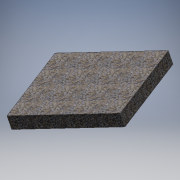
# Autodesk Inventor part: BaseMini
Saved by Autodesk Inventor 2016 (Build 200138000, 138)
## iProperties
Created: 2015-08-01
Part Number: BaseMini
Material: Concrete
Document SubType Name: Modeling
Designer: myhome
Density: 2.40731 g/cm^3
Appearance: Exposed Aggregate - Coarse
Mass: 134809 g
Surface Area: 14200 cm^2
Volume: 56000 cm^3
Author: myhome
Autodesk Inventor part; units mm, degrees
ref_plane "YZ Plane" through (0, 0, 0) normal (1, 0, 0) x (0, 1, 0)
ref_plane "XZ Plane" through (0, 0, 0) normal (0, 1, 0) x (-1, 0, 0)
ref_plane "XY Plane" through (0, 0, 0) normal (0, 0, 1) x (1, 0, 0)
sketch "Sketch5" plane through (0, 0, 0) normal (0, 0, 1) x (1, 0, 0)
  line L0 (0, 0) -> (800, 0)
  line L1 (800, 0) -> (800, 700)
  line L2 (800, 700) -> (0, 700)
  line L3 (0, 700) -> (0, 0)
  line L4 (800, 0) -> (800, 100)
  line L5 (800, 0) -> (800, 20)
  line L6 (800, 20) -> (800, 120)
  line L7 (800, 120) -> (700, 120) construction
  line L8 (700, 120) -> (700, 20) construction
  line L9 (700, 20) -> (800, 20) construction
  line L10 (0, 0) -> (0, 20) construction
  line L11 (0, 20) -> (0, 120) construction
  line L12 (0, 120) -> (100, 120) construction
  line L13 (100, 120) -> (100, 20) construction
  line L14 (100, 20) -> (0, 20) construction
  line L15 (0, 700) -> (0, 680) construction
  line L16 (0, 680) -> (100, 680) construction
  line L17 (100, 680) -> (100, 580) construction
  line L18 (100, 580) -> (0, 580) construction
  line L19 (0, 580) -> (0, 680) construction
  line L20 (800, 700) -> (800, 680) construction
  line L21 (800, 680) -> (700, 680) construction
  line L22 (700, 680) -> (700, 580) construction
  line L23 (700, 580) -> (800, 580) construction
  circle A0 centre (50, 70) radius 50
  circle A1 centre (750, 70) radius 50
  circle A2 centre (50, 630) radius 50
  circle A3 centre (750, 630) radius 50
  dimension "d12" = 800
  dimension "d13" = 700
  dimension "d18" = 20
  dimension "d19" = 100
  dimension "d20" = 100
  dimension "d21" = 100
  dimension "d22" = 100
  dimension "d23" = 20
  dimension "d24" = 100
  dimension "d25" = 100
  dimension "d26" = 100
  dimension "d27" = 100
  dimension "d28" = 20
  dimension "d29" = 100
  dimension "d30" = 100
  dimension "d31" = 100
  dimension "d32" = 100
  dimension "d33" = 20
  dimension "d34" = 100
  dimension "d35" = 100
  dimension "d36" = 100
  constraints: 48 end point, 9 perpendicular, 9 point on line, 4 centre point, 3 parallel, 1 horizontal
  measures "d12" distance of L1.end L2.end
  measures "d13" distance of L0.end L1.end
  measures "d18" distance of L0.end L5.end
  measures "d19" distance of L5.end L6.end
  measures "d20" distance of L6.end L7.end
  measures "d21" distance of L7.end L8.end
  measures "d22" distance of L8.end L5.end
  measures "d23" distance of L0.start L10.end
  measures "d24" distance of L10.end L11.end
  measures "d25" distance of L11.end L12.end
  measures "d26" distance of L12.end L13.end
  measures "d27" distance of L13.end L10.end
  measures "d28" distance of L2.end L15.end
  measures "d29" distance of L15.end L16.end
  measures "d30" distance of L16.end L17.end
  measures "d31" distance of L17.end L18.end
  measures "d32" distance of L18.end L15.end
  measures "d33" distance of L1.end L20.end
  measures "d34" distance of L20.end L21.end
  measures "d35" distance of L21.end L22.end
  measures "d36" distance of L22.end L23.end
extrude "Extrusion4" add sketch "Sketch5" against normal blind 100 contours A1 | A3 | A2 | A0 | L3 L2 L1 L0
body "Solid2"
